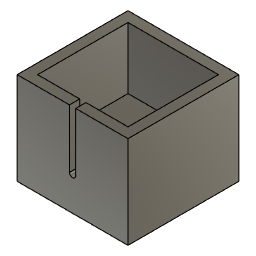
stamp_holder (Autodesk Fusion 360 design; units mm, degrees)
Autodesk Fusion 360 part; units mm, degrees
sketch "Sketch1" plane through (0, 0, 0) normal (0, 0, 1) x (1, 0, 0)
  line L0 (9, -9) -> (-9, -9)
  line L1 (-9, -9) -> (-9, 9)
  line L2 (-9, 9) -> (9, 9)
  line L3 (9, 9) -> (9, -9)
  line L4 (9, -9) -> (-9, 9) construction
  line L5 (-9, -9) -> (9, 9) construction
  dimension "d1" = 18
  constraint horizontal L0
  constraint perpendicular L0 L1
  constraint parallel L0 L2
  constraint parallel L1 L3
  constraint coincident L4 origin
  constraint coincident L5 origin
  constraint equal L1 L2
  measures "d1" distance of L1.end L2.end
extrude "Extrude1" add sketch "Sketch1" along normal blind 17
sketch "Sketch2" plane through (0, 0, 17) normal (0, 0, 1) x (-1, 0, 0)
  line L0 (-9, -9) -> (9, -9)
  line L1 (9, -9) -> (9, 9)
  line L2 (9, 9) -> (-9, 9)
  line L3 (-9, 9) -> (-9, -9)
  line L4 (-7.34, 7.34) -> (7.34, 7.34)
  line L5 (7.34, 7.34) -> (7.34, -7.34)
  line L6 (7.34, -7.34) -> (-7.34, -7.34)
  line L7 (-7.34, -7.34) -> (-7.34, 7.34)
  line L8 (-7.34, 7.34) -> (7.34, -7.34) construction
  line L9 (7.34, 7.34) -> (-7.34, -7.34) construction
  dimension "d4" = 14.68
  constraint horizontal L4
  constraint perpendicular L4 L5
  constraint parallel L4 L6
  constraint parallel L5 L7
  constraint coincident L8 origin
  constraint coincident L9 origin
  constraint equal L5 L6
  measures "d4" distance of L5.end L6.end
extrude "Extrude2" cut sketch "Sketch2" against normal blind 12 contours L4 L5 L6 L7
sketch "Sketch3" plane through (0, 0, 5) normal (0, 0, 1) x (-1, 0, 0)
  line L0 (-7.34, -7.34) -> (7.34, -7.34)
  line L1 (7.34, -7.34) -> (7.34, 7.34)
  line L2 (7.34, 7.34) -> (-7.34, 7.34)
  line L3 (-7.34, 7.34) -> (-7.34, -7.34)
  circle A0 centre (0, 0) radius 3.5
  dimension "d7" = 7
  constraint coincident A0.centre origin
  measures "d7" diameter of A0
extrude "Extrude3" cut sketch "Sketch3" against normal blind 3 contours A0
sketch "Sketch4" plane through (0, 0, 2) normal (0, 0, 1) x (-1, 0, 0)
  circle A0 centre (0, 0) radius 3.5
  circle A1 centre (0, 0) radius 1.85
  dimension "d10" = 3.7
  constraint coincident A0.centre A1.centre
  measures "d10" diameter of A1
extrude "Extrude4" cut sketch "Sketch4" against normal blind 2 contours A1
sketch "Sketch5" plane through (0, -9, 0) normal (0, -1, 0) x (1, 0, 0)
  line L0 (-9, 0) -> (9, 0)
  line L1 (9, 0) -> (9, 17)
  line L2 (9, 17) -> (-9, 17)
  line L3 (-9, 17) -> (-9, 0)
  line L4 (-9, 17) -> (9, 17)
  line L5 (9, 17) -> (9, 15)
  line L6 (9, 15) -> (-9, 15)
  line L7 (-9, 15) -> (-9, 17)
  line L8 (-9, 5) -> (9, 5) construction
  dimension "d14" = 5
  dimension "d16" = 10
  constraint horizontal L4
  constraint vertical L5
  constraint horizontal L6
  constraint vertical L7
  constraint coincident L1 L5.end
  constraint coincident L2.end L3.start
  constraint coincident L3 L8.start
  constraint coincident L1 L8.end
  constraint perpendicular L1 L8
  measures "d14" distance of L0 L8
  measures "d16" distance of L6 L8
extrude "Extrude5" cut sketch "Sketch5" against normal blind 18 contours L1 L2 L3 L4 L5 L6 L7
sketch "Sketch6" plane through (0, -9, 0) normal (0, -1, 0) x (1, 0, 0)
  line L0 (9, 15) -> (-9, 15)
  line L1 (-9, 15) -> (-9, 0)
  line L2 (-9, 0) -> (9, 0)
  line L3 (9, 0) -> (9, 15)
  line L4 (-0.5, 15) -> (-0.5, 5.5)
  arc A0 (-0.5, 5.5) -> (0.5, 5.5) centre (0, 5.5) ccw
  line L5 (0.5, 5.5) -> (0.5, 15)
  line L6 (-9, 5) -> (9, 5) construction
  dimension "d19" = 5
  dimension "d20" = 1
  constraint coincident L0 L4.start
  constraint perpendicular L0 L4
  constraint tangent L4 A0
  constraint coincident L0 L5.end
  constraint tangent A0 L5
  constraint perpendicular L0 L5
  constraint coincident L1 L6.start
  constraint coincident L3 L6.end
  constraint perpendicular L3 L6
  constraint tangent A0 L6
  constraint vertical origin A0.centre
  measures "d19" distance of L2 L6
  measures "d20" distance of L4 L5
extrude "Extrude6" cut sketch "Sketch6" against normal blind 1.66 contours L0 L4 A0 L5
